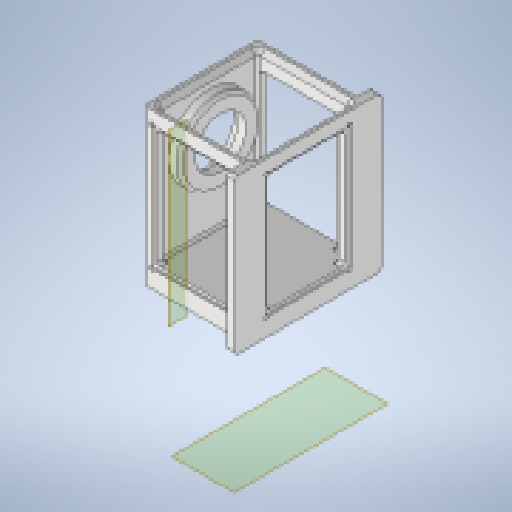
# Autodesk Inventor part: cuvette-w70mm-slide50x75mm-v1
Saved by Autodesk Inventor 2024 (Build 280153000, 153)
## iProperties
Created: 2025-09-30
Part Number: cuvette-w70mm-slide50x75mm-v1
Material: Generic
Document SubType Name: Modeling
Designer: N.Vladimirov
Density: 1 g/cm^3
Appearance: Default
Author: N.Vladimirov
Autodesk Inventor part; units mm, degrees
ref_plane "YZ Plane" through (0, 0, 0) normal (1, 0, 0) x (0, 1, 0)
ref_plane "XZ Plane" through (0, 0, 0) normal (0, 1, 0) x (-1, 0, 0)
ref_plane "XY Plane" through (0, 0, 0) normal (0, 0, 1) x (1, 0, 0)
sketch "Sketch1" plane through (0, 0, 0) normal (0, 0, 1) x (1, 0, 0)
  line L0 (30.5, -35) -> (-30.5, -35)
  line L1 (-30.5, -35) -> (-30.5, 35)
  line L2 (-30.5, 35) -> (30.5, 35)
  line L3 (30.5, 35) -> (30.5, -35)
  line L4 (30.5, -35) -> (-30.5, 35) construction
  line L5 (-30.5, -35) -> (30.5, 35) construction
  point P0 (0, 0)
  dimension "d0" = 61
  dimension "d1" = 70
  constraints: 12 end point, 2 midpoint, 2 parallel, 1 horizontal, 1 perpendicular
  measures "d0" distance of L1.end L2.end
  measures "d1" distance of L0.end L1.end
extrude "Extrusion1" add sketch "Sketch1" along normal blind 95.25
sketch "Sketch2" plane through (30.5, -35, 0) normal (1, 0, 0) x (0, 0, -1)
  line L0 (0, 0) -> (0, 70) projected
  line L1 (0, 70) -> (-95.25, 70) projected
  line L2 (-95.25, 0) -> (-95.25, 70) projected
  line L3 (0, 0) -> (-95.25, 0) projected
  line L4 (0, 70) -> (-95.25, 70) projected
  line L5 (-95.25, 70) -> (0, 70)
  line L6 (0, 70) -> (0, 80)
  line L7 (0, 80) -> (-95.25, 80)
  line L8 (-95.25, 80) -> (-95.25, 70)
  line L9 (-95.25, 70) -> (-95.25, 0) projected
  line L10 (-95.25, 0) -> (0, 0)
  line L11 (0, 0) -> (0, -10)
  line L12 (0, -10) -> (-95.25, -10)
  line L13 (-95.25, -10) -> (-95.25, 0)
  point P0 (0, 35)
  dimension "d4" = 10
  dimension "d5" = 10
  constraints: 16 end point, 4 parallel, 2 horizontal, 2 perpendicular, 1 point on line
  measures "d4" distance of L6.end L5.end
  measures "d5" distance of L10.end L11.end
extrude "Extrusion2" add sketch "Sketch2" along normal blind 5
sketch "Sketch12" plane through (35.5, -35, 0) normal (1, 0, 0) x (0, 0, -1)
  line L0 (-83.021, 9.25) -> (-9.5, 9.25)
  line L1 (-8, 10.75) -> (-8, 59.25)
  line L2 (-9.5, 60.75) -> (-83.021, 60.75)
  line L3 (-84.5, 59.5) -> (-84.5, 11)
  line L4 (-10, 56.75) -> (-10, 13.25)
  line L5 (-12, 11.25) -> (-80.5, 11.25)
  line L6 (-82.5, 13.25) -> (-82.5, 56.75)
  line L7 (-80.5, 58.75) -> (-12, 58.75)
  line L8 (0, -10) -> (0, 80) projected
  arc A0 (-10, 56.75) -> (-12, 58.75) centre (-12, 56.75) ccw
  arc A1 (-12, 11.25) -> (-10, 13.25) centre (-12, 13.25) ccw
  arc A2 (-82.5, 13.25) -> (-80.5, 11.25) centre (-80.5, 13.25) ccw
  arc A3 (-80.5, 58.75) -> (-82.5, 56.75) centre (-80.5, 56.75) ccw
  arc A4 (-8, 59.25) -> (-9.5, 60.75) centre (-8, 60.75) ccw
  arc A5 (-9.5, 9.25) -> (-8, 10.75) centre (-8, 9.25) ccw
  arc A6 (-83.021, 60.75) -> (-84.5, 59.5) centre (-84.5, 61) ccw
  arc A7 (-84.5, 11) -> (-83.021, 9.25) centre (-84.5, 9.5) ccw
  line L9 (0, 35) -> (-110.0583, 35)
  point P0 (0, -8)
  point P1 (0, 78)
  dimension "d57" = 2
  dimension "d58" = 8
  dimension "d59" = 2
  dimension "d60" = 3
  dimension "d61" = 3
  dimension "d62" = 3
  dimension "d63" = 3
  dimension "d119" = 2
  dimension "d120" = 76.5
  dimension "d121" = 51.5
  dimension "d122" = 2
  dimension "d123" = 2
  constraints: 18 end point, 16 point on circle, 8 centre point, 8 tangent, 4 parallel, 3 equal radius, 2 horizontal, 2 perpendicular, 1 other
  measures "d57" distance between parallel lines of L1 L4
  measures "d58" distance between parallel lines of L1 L8
  measures "d59" radius of A0
  measures "d60" diameter of A4
  measures "d61" diameter of A5
  measures "d62" diameter of A6
  measures "d63" diameter of A7
  measures "d119" distance between parallel lines of L3 L6
  measures "d120" distance between parallel lines of L3 L1
  measures "d121" distance between parallel lines of L0 L2
  measures "d122" distance between parallel lines of L7 L2
  measures "d123" distance between parallel lines of L5 L0
sketch "Sketch13" plane through (-30.5, -35, 0) normal (-1, 0, 0) x (0, 0, 1)
  line L0 (8, 10.75) -> (8, 59.25) projected
  line L1 (10, 56.75) -> (10, 13.25) projected
  line L2 (83.021, 9.25) -> (9.5, 9.25) projected
  arc A0 (8, 10.75) -> (9.5, 9.25) centre (8, 9.25) ccw projected
  line L3 (12, 11.25) -> (80.5, 11.25) projected
  arc A1 (10, 13.25) -> (12, 11.25) centre (12, 13.25) ccw projected
  arc A2 (9.5, 60.75) -> (8, 59.25) centre (8, 60.75) ccw projected
  line L4 (9.5, 60.75) -> (83.021, 60.75) projected
  line L5 (80.5, 58.75) -> (12, 58.75) projected
  line L6 (84.5, 59.5) -> (84.5, 11) projected
  line L7 (82.5, 13.25) -> (82.5, 56.75) projected
  arc A3 (84.5, 59.5) -> (83.021, 60.75) centre (84.5, 61) ccw projected
  arc A4 (83.021, 9.25) -> (84.5, 11) centre (84.5, 9.5) ccw projected
  arc A5 (80.5, 11.25) -> (82.5, 13.25) centre (80.5, 13.25) ccw projected
  arc A6 (82.5, 56.75) -> (80.5, 58.75) centre (80.5, 56.75) ccw projected
  arc A7 (12, 58.75) -> (10, 56.75) centre (12, 56.75) ccw projected
  point P0 (0, 35)
extrude "Extrusion12" cut sketch "Sketch12" against normal blind 20 contours L9 L4 A1 L5 A2 L6 | L6 A3 L7 A0 L4 L9
ref_plane "LightSheet Plane1" through (-5.1, -35, 0) normal (-1, 0, 0) x (0, 0, 1)
sketch "Sketch15" plane through (-30.5, 35, 95.25) normal (0, 1, 0) x (1, 0, 0)
  line L0 (54.25, 10.75) -> (6.25, 10.75)
  line L1 (4.75, 12.25) -> (4.75, 85.75)
  line L2 (6.25, 87.25) -> (54.75, 87.25)
  line L3 (56.25, 85.75) -> (56.25, 12.1642)
  line L4 (61, 95.25) -> (0, 95.25) projected
  line L5 (52.25, 85.25) -> (8.75, 85.25)
  line L6 (6.75, 83.25) -> (6.75, 14.75)
  line L7 (8.75, 12.75) -> (52.25, 12.75)
  line L8 (54.25, 14.75) -> (54.25, 83.25)
  arc A0 (8.75, 85.25) -> (6.75, 83.25) centre (8.75, 83.25) ccw
  arc A1 (54.25, 83.25) -> (52.25, 85.25) centre (52.25, 83.25) ccw
  arc A2 (52.25, 12.75) -> (54.25, 14.75) centre (52.25, 14.75) ccw
  arc A3 (6.75, 14.75) -> (8.75, 12.75) centre (8.75, 14.75) ccw
  arc A4 (6.25, 87.25) -> (4.75, 85.75) centre (4.75, 87.25) ccw
  arc A5 (56.25, 85.75) -> (54.75, 87.25) centre (56.25, 87.25) ccw
  arc A6 (54.25, 10.75) -> (56.25, 12.1642) centre (55.75, 10.75) ccw
  arc A7 (4.75, 12.25) -> (6.25, 10.75) centre (4.75, 10.75) ccw
  line L9 (30.5, 95.25) -> (30.5, -2.0422)
  dimension "d84" = 8
  dimension "d85" = 2
  dimension "d86" = 2
  dimension "d87" = 3
  dimension "d88" = 3
  dimension "d89" = 3
  dimension "d90" = 3
  dimension "d124" = 51.5
  dimension "d125" = 76.5
  dimension "d126" = 2
  dimension "d127" = 2
  dimension "d128" = 2
  constraints: 18 end point, 16 point on circle, 8 centre point, 8 tangent, 4 parallel, 3 equal radius, 2 perpendicular, 1 horizontal, 1 vertical, 1 other
  measures "d84" distance between parallel lines of L2 L4
  measures "d85" distance between parallel lines of L2 L5
  measures "d86" radius of A0
  measures "d87" diameter of A4
  measures "d88" diameter of A5
  measures "d89" diameter of A6
  measures "d90" diameter of A7
  measures "d124" distance between parallel lines of L3 L1
  measures "d125" distance between parallel lines of L0 L2
  measures "d126" distance between parallel lines of L0 L7
  measures "d127" distance between parallel lines of L6 L1
  measures "d128" distance between parallel lines of L8 L3
extrude "Extrusion16" cut sketch "Sketch15" against normal through all contours L9 L5 A1 L8 A2 L7 | L7 A3 L6 A0 L5 L9
sketch "Sketch16" plane through (-30.5, -35, 0) normal (0, -1, 0) x (1, 0, 0)
  line L0 (6.25, 8) -> (54.75, 8) projected
  arc A0 (4.75, 9.5) -> (6.25, 8) centre (4.75, 8) ccw projected
  line L1 (4.75, 83) -> (4.75, 9.5) projected
  arc A1 (54.75, 8) -> (56.25, 9.5) centre (56.25, 8) ccw projected
  line L2 (56.25, 9.5) -> (56.25, 83.0858) projected
  arc A2 (56.25, 83.0858) -> (54.25, 84.5) centre (55.75, 84.5) ccw projected
  line L3 (54.25, 84.5) -> (6.25, 84.5) projected
  arc A3 (6.25, 84.5) -> (4.75, 83) centre (4.75, 84.5) ccw projected
  point P0 (30.5, 0)
extrude "Extrusion17" cut sketch "Sketch16" against normal blind 1.5
sketch "Sketch17" plane through (0, 0, 0) normal (0, 0, -1) x (-1, 0, 0)
  line L0 (25.5, 30) -> (-30.5, 30)
  line L1 (-30.5, 30) -> (-30.5, -30)
  line L2 (-30.5, -30) -> (25.5, -30)
  line L3 (25.5, -30) -> (25.5, 30)
  line L4 (-30.5, 35) -> (30.5, 35) projected
  line L5 (30.5, 35) -> (30.5, -35) projected
  line L6 (30.5, -35) -> (-30.5, -35) projected
  line L7 (-30.5, 35) -> (-30.5, 45) projected
  point P0 (0, 0)
  dimension "d95" = 5
  dimension "d96" = 5
  dimension "d97" = 5
  dimension "d98" = 0
  constraints: 8 end point, 2 parallel, 1 horizontal, 1 perpendicular
  measures "d95" distance between parallel lines of L0 L4
  measures "d96" distance between parallel lines of L3 L5
  measures "d97" distance between parallel lines of L6 L2
  measures "d98" distance between parallel lines of L7 L1
extrude "Extrusion18" cut sketch "Sketch17" against normal up to surface (82.5 mm away)
fillet "Fillet2" radius 1.5 11 edges at (30.5, 25.875, 82.5) (26.125, 30, 82.5) (30.5, 30, 41.25) (30.5, -30, 41.25) (26.125, -30, 82.5) (30.5, -25.875, 82.5) (-25.5, -30, 41.25) (-25.5, 30, 41.25) (-25.5, 0, 82.5) (-23.625, 30, 82.5) (-23.625, -30, 82.5)
extrude "Extrusion19" cut sketch "Sketch15" against normal blind 1.5
fillet "Fillet3" radius 2 4 edges at (33, 45, 0) (33, 45, 95.25) (33, -45, 0) (33, -45, 95.25)
extrude "Extrusion20" cut sketch "Sketch12" against normal blind 1.5
sketch "Sketch18" plane through (0, 0, 95.25) normal (0, 0, 1) x (1, 0, 0)
  point P0 (0, 0)
  point P1 (0, 0)
  constraints: 1 coincident
hole "Hole2" at (0, 0, 95.25) direction (0, 0, -1) diameter 5.588 depth 10 tip angle 118 thread size "1/4-36 UNS" class "2B" standard "ANSI Unified Screw Threads"
sketch "Sketch19" plane through (-30.5, 35, 95.25) normal (0, 1, 0) x (1, 0, 0)
  circle A0 centre (30.5, 0) radius 0.5
  point P0 (30.5, 95.25)
  dimension "d116" = 1
  constraints: 1 centre point, 1 coincident
  measures "d116" diameter of A0
extrude "Extrusion22" cut sketch "Sketch19" against normal through all
chamfer "Chamfer1" distance 3 angle 45 8 edges at (-25.5, 0, 0) (-25.0607, -29.5607, 0) (2.5, -30, 0) (30.0607, -29.5607, 0) (30.5, 0, 0) (30.0607, 29.5607, 0) (2.5, 30, 0) (-25.0607, 29.5607, 0)
fillet "Fillet4" radius 2 2 edges at (-30.5, 35, 47.625) (-30.5, -35, 47.625)
ref_plane "Benchtop-Baseplate" through (0, 0, 166.25) normal (0, 0, 1) x (1, 0, 0)
sketch "Sketch21" plane through (-30.5, -33, 0) normal (-1, 0, 0) x (0, 0, 1)
  circle A0 centre (31.25, 33) radius 21
  line L0 (166.25, 96) -> (166.25, -30) projected
  circle A1 centre (31.25, 33) radius 15.5
  circle A2 centre (31.25, 33) radius 25
  point P0 (0, 33)
  dimension "d134" = 42
  dimension "d135" = 135
  dimension "d136" = 31
  dimension "d137" = 50
  constraints: 3 centre point, 2 coincident
  measures "d134" diameter of A0
  measures "d135" distance from line of L0 A0.centre
  measures "d136" diameter of A1
  measures "d137" diameter of A2
extrude "Extrusion23" add sketch "Sketch21" against normal blind 12 contours A0 | A1 | A2
fillet "Fillet5" radius 2 1 edges at (-18.5, 0, 6.25)
extrude "Extrusion24" cut sketch "Sketch21" against normal blind 7 contours A0
extrude "Extrusion25" cut sketch "Sketch21" against normal up to surface (12 mm away) contours A1
sketch "Sketch22" plane through (-30.5, -33, 0) normal (-1, 0, 0) x (0, 0, 1)
  circle A0 centre (87.75, 7.5) radius 3.3 projected
  circle A1 centre (87.75, 58.5) radius 3.3 projected
  point P0 (0, 33)
hole "Hole3" at (-30.5, -25.5, 87.75) at (-30.5, 25.5, 87.75) direction (1, 0, 0) diameter 4.917 depth 25 tip angle 118 thread size "M6x1" class "6H" standard "ISO Metric profile"
body "Solid1"
